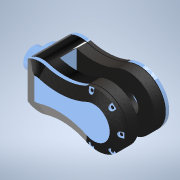
# Autodesk Inventor part: Part5
Saved by Autodesk Inventor 2022 (Build 260153000, 153)
## iProperties
Created: 2023-11-30
Part Number: Part5
Material: Generic
Document SubType Name: Modeling
Designer: harshidd
Density: 1 g/cm^3
Appearance: Red
Author: harshidd
Autodesk Inventor part; units mm, degrees
ref_plane "XZ Plane" through (0, 0, 0) normal (0, 1, 0) x (-1, 0, 0)
ref_plane "XY Plane" through (0, 0, 0) normal (0, 0, 1) x (1, 0, 0)
sketch "Sketch1" plane through (0, 0, 0) normal (0, 0, 1) x (1, 0, 0)
  circle A0 centre (0, 0) radius 27.5
  dimension "d0" = 55
  constraints: 1 centre point, 1 coincident
  measures "d0" diameter of A0
extrude "Extrusion1" add sketch "Sketch1" along normal blind 5
ref_plane "Work Plane1" through (-27.5, 0, 0) normal (1, 0, 0) x (0, 1, 0)
sketch "Sketch2" plane through (-27.5, 0, 0) normal (1, 0, 0) x (0, 1, 0)
  line L0 (0, 0) -> (0, 150) construction
  line L1 (0, 0) -> (0, 23)
  line L2 (27.5, 5) -> (-27.5, 5) projected
  line L3 (0, 150) -> (0, 110)
  arc A0 (36.1578, 92.8941) -> (-36.1578, 92.8941) centre (0, 110) ccw
  arc A1 (36.1578, 92.8941) -> (31.5081, 32.3537) centre (112.9932, 56.5441) ccw
  arc A2 (-31.5081, 32.3537) -> (-36.1578, 92.8941) centre (-112.9932, 56.5441) ccw
  line L4 (27.5, 5) -> (-27.5, 5)
  arc A3 (-31.5081, 32.3537) -> (-27.5, 5) centre (0, 23) ccw
  arc A4 (27.5, 5) -> (31.5081, 32.3537) centre (0, 23) ccw
  dimension "d4" = 150
  dimension "d5" = 23
  dimension "d6" = 40
  dimension "d7" = 85
  constraints: 11 point on circle, 8 end point, 5 centre point, 3 symmetric about line, 2 coincident, 2 point on line, 1 collinear, 1 tangent, 1 vertical, 1 other
  measures "d4" distance of L0.start L0.end
  measures "d5" distance of L0.start L1.end
  measures "d6" distance of L0.end L3.end
  measures "d7" radius of A1
extrude "Extrusion2" add sketch "Sketch2" along normal blind 15
sketch "Sketch3" plane through (-27.5, 0, 0) normal (-1, 0, 0) x (0, 0, 1)
  arc A0 (92.8941, -36.1578) -> (92.8941, 36.1578) centre (110, 0) ccw projected
  arc A1 (32.3537, 31.5081) -> (92.8941, 36.1578) centre (56.5441, 112.9932) ccw projected
  arc A2 (32.3537, 31.5081) -> (5, 27.5) centre (23, 0) ccw projected
  line L0 (5, 0) -> (5, 27.5) projected
  line L1 (5, -27.5) -> (5, 0) projected
  arc A3 (5, -27.5) -> (32.3537, -31.5081) centre (23, 0) ccw projected
  arc A4 (92.8941, -36.1578) -> (32.3537, -31.5081) centre (56.5441, -112.9932) ccw projected
  arc A5 (93.7494, -34.3499) -> (93.7494, 34.3499) centre (110, 0) ccw
  arc A6 (93.7494, -34.3499) -> (31.7845, -29.5908) centre (56.5441, -112.9932) ccw
  arc A7 (7, -26.3966) -> (31.7845, -29.5908) centre (23, 0) ccw
  line L2 (7, -26.3966) -> (7, 0)
  line L3 (7, 0) -> (7, 26.3966)
  arc A8 (31.7845, 29.5908) -> (7, 26.3966) centre (23, 0) ccw
  arc A9 (31.7845, 29.5908) -> (93.7494, 34.3499) centre (56.5441, 112.9932) ccw
  point P0 (0, 0)
  dimension "d10" = 2
  constraints: 10 point on circle, 5 centre point, 4 end point, 6 other
  measures "d10" radial gap between concentric circles of A1 A9
extrude "Extrusion3" add sketch "Sketch3" along normal blind 1 contours A6 A7 L2 L3 A8 A9 A5
sketch "Sketch4" plane through (-28.5, 0, 0) normal (-1, 0, 0) x (0, 0, 1)
  arc A0 (92.8941, -36.1578) -> (92.8941, 36.1578) centre (110, 0) ccw projected
  arc A1 (32.3537, 31.5081) -> (92.8941, 36.1578) centre (56.5441, 112.9932) ccw projected
  arc A2 (32.3537, 31.5081) -> (5, 27.5) centre (23, 0) ccw projected
  line L0 (5, 0) -> (5, 27.5) projected
  line L1 (5, -27.5) -> (5, 0) projected
  arc A3 (5, -27.5) -> (32.3537, -31.5081) centre (23, 0) ccw projected
  arc A4 (92.8941, -36.1578) -> (32.3537, -31.5081) centre (56.5441, -112.9932) ccw projected
  point P0 (0, 0)
extrude "Extrusion4" add sketch "Sketch4" along normal blind 5
ref_plane "Work Plane2" through (-39.5, 0, 0) normal (-1, 0, 0) x (0, 0, 1)
sketch "Sketch5" plane through (-39.5, 0, 0) normal (-1, 0, 0) x (0, 0, 1)
  arc A0 (99.7365, -21.6947) -> (99.7365, 21.6947) centre (110, 0) ccw
  arc A1 (99.7365, -21.6947) -> (27.8003, -16.1697) centre (56.5441, -112.9932) ccw
  arc A2 (21, -16.7482) -> (27.8003, -16.1697) centre (23, 0) ccw
  line L0 (21, -16.7482) -> (21, 16.7482)
  arc A3 (27.8003, 16.1697) -> (21, 16.7482) centre (23, 0) ccw
  arc A4 (27.8003, 16.1697) -> (99.7365, 21.6947) centre (56.5441, 112.9932) ccw
  point P0 (0, 0)
  constraints: 10 point on circle, 5 centre point, 2 end point
loft "Loft1" add profiles "Sketch5" section 1 edges at (-33.5, 0, 150) (-33.5, 28.2428, 63.0533) (-33.5, 32.5199, 18.235) (-33.5, 0, 5) (-33.5, -32.5199, 18.235) (-33.5, -28.2428, 63.0533)
ref_plane "Work Plane3" through (-33.5, 27.5, 5) normal (1, 0, 0) x (0, 1, 0)
sketch "Sketch6" plane through (-33.5, 27.5, 5) normal (1, 0, 0) x (0, 1, 0)
  line L0 (-27.5, 145) -> (-27.5, 141) construction
  line L1 (-23.5, 144.7995) -> (-23.5, 141)
  line L2 (-31.5, 144.7995) -> (-31.5, 141)
  arc A0 (-31.5, 141) -> (-23.5, 141) centre (-27.5, 141) ccw
  arc A1 (-23.5, 144.7995) -> (-31.5, 144.7995) centre (-27.5, 105) ccw
  point P0 (-27.5, -5)
  dimension "d21" = 4
  dimension "d22" = 4
  dimension "d23" = 4
  constraints: 6 end point, 5 point on circle, 2 centre point, 2 parallel, 1 coincident, 1 vertical
  measures "d21" distance of L0.start L0.end
  measures "d22" distance between parallel lines of L0 L1
  measures "d23" distance between parallel lines of L0 L2
extrude "Extrusion5" cut sketch "Sketch6" against normal blind 5
sketch "Sketch7" plane through (-33.5, 27.5, 5) normal (-1, 0, 0) x (0, 0, 1)
  arc A0 (141, -23.5) -> (141, -31.5) centre (141, -27.5) ccw projected
  circle A1 centre (141, -27.5) radius 1.25
  circle A2 centre (141, -27.5) radius 2.25
  point P0 (-5, -27.5)
  dimension "d26" = 2.5
  dimension "d27" = 1
  constraints: 2 centre point, 1 coincident
  measures "d26" diameter of A1
  measures "d27" radial gap between concentric circles of A1 A2
extrude "Extrusion6" add sketch "Sketch7" along normal blind 0.5
pattern_circular "Circular Pattern1" count 7 over 360 about axis through (-33.5, 0, 110) along (-1, 0, 0) of "Extrusion5", "Extrusion6" skipped copies 4 5
sketch "Sketch8" plane through (-12.5, 0, 0) normal (1, 0, 0) x (0, 0, -1)
  arc A0 (-5, 27.5) -> (-32.3537, 31.5081) centre (-23, 0) ccw projected
  line L0 (-5, 27.5) -> (-5, -27.5) projected
  arc A1 (-32.3537, -31.5081) -> (-5, -27.5) centre (-23, 0) ccw projected
  line L1 (-32.3537, 31.5081) -> (-32.3537, -31.5081)
  point P0 (0, 0)
  point P1 (-5, -24.4949)
  point P2 (-5, 24.4949)
  constraints: 2 end point, 1 vertical
extrude "Extrusion7" add sketch "Sketch8" along normal up to surface (40 mm away)
sketch "Sketch9" plane through (-12.5, 0, 0) normal (1, 0, 0) x (0, 0, -1)
  arc A0 (-99.7365, 21.6947) -> (-99.7365, -21.6947) centre (-110, 0) ccw projected
  circle A1 centre (-110, 0) radius 15
  point P0 (0, 0)
  dimension "d35" = 30
  constraints: 1 centre point, 1 coincident
  measures "d35" diameter of A1
extrude "Extrusion8" cut sketch "Sketch9" against normal blind 20
mirror "Mirror1" about plane through (0, 0, 0) normal (1, 0, 0) of "Extrusion2", "Extrusion3", "Extrusion4", "Loft1", "Extrusion5", "Extrusion6", "Circular Pattern1", "Extrusion7", "Extrusion8"
sketch "Sketch10" plane through (0, 0, 0) normal (0, 0, -1) x (-1, 0, 0)
  circle A0 centre (0, 0) radius 15
  dimension "d38" = 30
  constraints: 1 centre point, 1 coincident
  measures "d38" diameter of A0
extrude "Extrusion9" add sketch "Sketch10" along normal blind 20
ref_plane "Work Plane4" through (39.5, 0, 0) normal (-1, 0, 0) x (0, 0, 1)
ref_plane "Work Plane5" through (33.5, 27.5, 5) normal (1, 0, 0) x (0, 1, 0)
body "Solid1"
